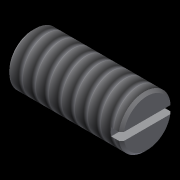
# Autodesk Inventor part: Screw1G
Saved by Autodesk Inventor 2020 (Build 240168000, 168)
## iProperties
Created: 2018-03-10
Part Number: Screw1G
Document SubType Name: Modeling
Designer: Administrator
Density: 1 g/cm^3
Mass: 0.00169079 g
Surface Area: 0.0863077 cm^2
Volume: 0.00169079 cm^3
Material: 一般
Appearance: 預設
Author: Administrator
Autodesk Inventor part; units mm, degrees
ref_plane "YZ Plane" through (0, 0, 0) normal (1, 0, 0) x (0, 1, 0)
ref_plane "XZ Plane" through (0, 0, 0) normal (0, 1, 0) x (-1, 0, 0)
ref_plane "XY Plane" through (0, 0, 0) normal (0, 0, 1) x (1, 0, 0)
sketch "Sketch1" plane through (0, 0, 0) normal (0, 0, 1) x (1, 0, 0)
  line L0 (0, 0) -> (2.2, 0)
  line L1 (2.2, 0.5) -> (0, 0.5)
  line L2 (0, 0) -> (0, 0.5)
  line L3 (0, 0) -> (2.2, 0) construction
  line L4 (2.2, 0.5) -> (2.2, 0)
  dimension "d25" = 0.5
  dimension "d43" = 2.2
  constraints: 10 end point, 1 perpendicular, 1 other
  measures "d25" distance between parallel lines of L1 L0
  measures "d43" distance of L1.start L1.end
revolve "Revolution1" add sketch "Sketch1" angle 360 about axis through (0, 0, 0) along (1, 0, 0)
chamfer "Chamfer1" distance 0.05 angle 45 2 edges at (0, -0.5, 0) (2.2, -0.5, 0)
thread "Thread4" size "M1x0.25" class "6g" standard "ANSI Metric M Profile" full length
sketch "Sketch4" plane through (2.2, 0, 0) normal (1, 0, 0) x (0, 0, -1)
  circle A0 centre (0, 0) radius 0.45 projected
  line L0 (-0.075, 0.7107) -> (0.075, 0.7107)
  line L1 (0.075, 0.7107) -> (0.075, -0.5992)
  line L2 (0.075, -0.5992) -> (-0.075, -0.5992)
  line L3 (-0.075, -0.5992) -> (-0.075, 0.7107)
  dimension "d46" = 0.15
  dimension "d47" = 0.075
  constraints: 8 end point, 2 parallel, 1 horizontal, 1 perpendicular
  measures "d46" distance of L0.start L0.end
  measures "d47" distance from line of L1 A0.centre
extrude "Extrusion3" cut sketch "Sketch4" against normal blind 0.2 contours L1 A0 L3 | A0 L3 L0 L1 | L1 L2 L3 A0
